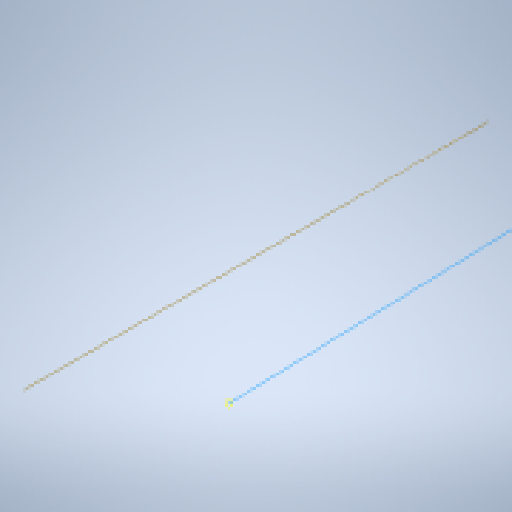
# Autodesk Inventor part: laserbeam1
Saved by Autodesk Inventor 2023 (Build 270158000, 158)
## iProperties
Created: 2024-05-16
Part Number: laserbeam1
Material: Generic
Document SubType Name: Modeling
Designer: kerlin
Density: 1 g/cm^3
Appearance: Default
Author: kerlin
Autodesk Inventor part; units mm, degrees
ref_plane "YZ Plane" through (0, 0, 0) normal (1, 0, 0) x (0, 1, 0)
sketch "Sketch1" plane through (0, 0, 0) normal (0, 0, 1) x (1, 0, 0)
  circle A0 centre (0, 0) radius 0.3175
  dimension "d0" = 0.635
  constraints: 1 centre point, 1 coincident
  measures "d0" diameter of A0
ref_plane "Work Plane1" through (-17.2208, -17.2208, 280) normal (0, 0, -1) x (0.3158, 0.9488, 0)
ref_plane "Work Plane2" through (-0.8039, -1.5491, 73.0001) normal (0.7059, 0.0418, -0.7071) x (-0.0591, 0.9983, 0)
extrude "Extrusion1" add sketch "Sketch1" along normal up to surface surface through (-0.8039, -1.5491, 73.0001) normal (0.7059, 0.0418, -0.7071)
body "Solid1"
